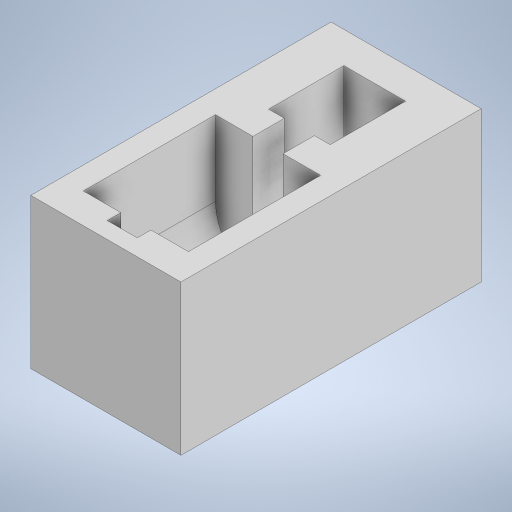
# Autodesk Inventor part: dcmotor_housing
Saved by Autodesk Inventor 2023 (Build 270158000, 158)
## iProperties
Created: 2023-03-20
Part Number: dcmotor_housing
Material: Generic
Document SubType Name: Modeling
Designer: caleb
Density: 1 g/cm^3
Appearance: Default
Author: caleb
Autodesk Inventor part; units mm, degrees
sketch "Sketch1" plane through (0, 0, 0) normal (0, 1, 0) x (-1, 0, 0)
  line L0 (0, 0) -> (50, 0)
  line L1 (50, 0) -> (50, -100)
  line L2 (50, -100) -> (0, -100)
  line L3 (0, -100) -> (0, 0)
  line L4 (25, 0) -> (25, -100)
  line L5 (7.5, -54) -> (7.5, -10)
  line L6 (7.5, -10) -> (42.5, -10)
  line L7 (42.5, -10) -> (42.5, -54)
  line L8 (42.5, -54) -> (7.5, -54)
  line L9 (7.5, -54) -> (42.5, -10) construction
  line L10 (7.5, -10) -> (42.5, -54) construction
  line L11 (7.5, -54) -> (51.5, -54) construction
  line L12 (14.75, -64.45) -> (14.75, -89.55)
  line L13 (14.75, -89.55) -> (35.25, -89.55)
  line L14 (35.25, -89.55) -> (35.25, -64.45)
  line L15 (35.25, -64.45) -> (14.75, -64.45)
  line L16 (14.75, -64.45) -> (35.25, -89.55) construction
  line L17 (14.75, -89.55) -> (35.25, -64.45) construction
  line L18 (14.75, -64.45) -> (39.85, -64.45) construction
  line L19 (25, -10) -> (25, -15)
  line L20 (25, -10) -> (30, -10) construction
  line L21 (20, -20) -> (30, -20)
  line L22 (30, -20) -> (30, -10)
  line L23 (30, -10) -> (20, -10)
  line L24 (20, -10) -> (20, -20)
  line L25 (20, -20) -> (30, -10) construction
  line L26 (30, -20) -> (20, -10) construction
  line L27 (20, -20) -> (30, -20) construction
  line L28 (30, -15) -> (20, -15)
  point P0 (25, -32)
  point P1 (25, -77)
  point P2 (25, -54)
  point P3 (25, -77)
  dimension "d0" = 50
  dimension "d1" = 100
  dimension "d4" = 44
  dimension "d5" = 90
  dimension "d6" = 35
  dimension "d7" = 10
  dimension "d8" = 25.1
  dimension "d9" = 90
  dimension "d10" = 20.5
  dimension "d35" = 5
  dimension "d36" = 90
  dimension "d37" = 0
  constraints: 58 end point, 11 midpoint, 9 parallel, 5 horizontal, 4 equal length, 4 perpendicular, 3 point on line, 1 coincident, 1 collinear, 1 vertical
  measures "d0" distance of L1.end L2.end
  measures "d1" distance of L0.end L1.end
  measures "d4" distance of L5.start L5.end
  measures "d5" angle of L11 L5
  measures "d6" distance of L5.end L6.end
  measures "d7" distance between parallel lines of L6 L0
  measures "d8" distance of L12.start L12.end
  measures "d9" angle of L12 L18
  measures "d10" distance of L13.end L12.end
  measures "d35" distance of L19.start L19.end
  measures "d36" angle of L19 L20
  measures "d37" distance between parallel lines of L21 L27
extrude "Extrusion1" add sketch "Sketch1" against normal blind 50
ref_plane "Work Plane3" through (-14.75, 0, -89.55) normal (0, 0, -1) x (-1, 0, 0)
ref_plane "Work Plane4" through (-7.5, 0, -54) normal (0, 0, -1) x (-1, 0, 0)
sketch "Sketch3" plane through (-14.75, 0, -89.55) normal (0, 0, -1) x (-1, 0, 0)
  line L0 (35.25, 0) -> (-14.75, 0) projected
  line L1 (35.25, 0) -> (35.25, -50) projected
  line L2 (-14.75, -50) -> (35.25, -50) projected
  line L3 (-14.75, 0) -> (-14.75, -50) projected
  circle A0 centre (10.25, -25) radius 10.1
  line L4 (20.35, -35.1) -> (20.35, -14.9)
  line L5 (20.35, -14.9) -> (0.15, -14.9)
  line L6 (0.15, -14.9) -> (0.15, -35.1)
  line L7 (0.15, -35.1) -> (20.35, -35.1)
  line L8 (20.35, -35.1) -> (0.15, -14.9) construction
  line L9 (20.35, -14.9) -> (0.15, -35.1) construction
  line L10 (20.35, -35.1) -> (40.55, -35.1) construction
  point P0 (10.25, -35.1)
  point P1 (0.15, -25)
  point P2 (20.35, -25)
  dimension "d18" = 20.2
  dimension "d21" = 90
  constraints: 14 end point, 2 midpoint, 2 parallel, 2 perpendicular, 1 centre point, 1 coincident, 1 horizontal
  measures "d18" diameter of A0
  measures "d21" angle of L10 L4
ref_plane "Work Plane5" through (-14.75, 0, -64.45) normal (0, 0, -1) x (-1, 0, 0)
ref_plane "Work Plane6" through (-7.5, 0, -10) normal (0, 0, -1) x (-1, 0, 0)
ref_plane "Work Plane7" through (-35.1, -35.1, -89.55) normal (0, 1, 0) x (1, 0, 0)
extrude "Extrusion5" cut sketch "Sketch1" against normal up to surface (35.1 mm away) contours L13 L12 L15 L4 | L4 L15 L14 L13
extrude "Extrusion6" add sketch "Sketch3" against normal up to surface (25.1 mm away) contours L4 L7 A0 | L7 L6 A0
sketch "Sketch4" plane through (-7.5, 0, -54) normal (0, 0, -1) x (-1, 0, 0)
  line L0 (42.5, 0) -> (-7.5, 0) projected
  line L1 (42.5, 0) -> (42.5, -50) projected
  line L2 (-7.5, -50) -> (42.5, -50) projected
  line L3 (-7.5, 0) -> (-7.5, -50) projected
  circle A0 centre (17.5, -25) radius 17.5
  line L4 (0, -42.5) -> (0, -7.5)
  line L5 (0, -7.5) -> (35, -7.5)
  line L6 (35, -7.5) -> (35, -42.5)
  line L7 (35, -42.5) -> (0, -42.5)
  line L8 (0, -42.5) -> (35, -7.5) construction
  line L9 (0, -7.5) -> (35, -42.5) construction
  line L10 (0, -42.5) -> (35, -42.5) construction
  point P0 (17.5, -42.5)
  point P1 (35, -25)
  point P2 (0, -25)
  dimension "d26" = 35
  dimension "d27" = 90
  constraints: 14 end point, 2 midpoint, 2 parallel, 2 perpendicular, 1 centre point, 1 coincident, 1 horizontal
  measures "d26" diameter of A0
  measures "d27" angle of L10 L4
ref_plane "Work Plane8" through (-7.5, -42.5, -54) normal (0, 1, 0) x (1, 0, 0)
extrude "Extrusion7" cut sketch "Sketch1" against normal up to surface (42.5 mm away) contours L6 L22 L28 L4 | L4 L28 L24 L6 | L28 L22 L21 L4 | L4 L21 L24 L28 | L24 L21 L4 L8 L5 L6 | L6 L7 L8 L4 L21 L22
extrude "Extrusion8" add sketch "Sketch4" against normal up to surface (44 mm away) contours L6 L7 A0 | L7 L4 A0
sketch "Sketch5" plane through (-14.75, 0, -64.45) normal (0, 0, -1) x (-1, 0, 0)
  line L0 (35.25, 0) -> (-14.75, 0) projected
  line L1 (35.25, 0) -> (35.25, -50) projected
  line L2 (-14.75, -50) -> (35.25, -50) projected
  line L3 (-14.75, 0) -> (-14.75, -50) projected
  circle A0 centre (10.25, -25) radius 5
  dimension "d32" = 10
  constraints: 1 centre point, 1 coincident
  measures "d32" diameter of A0
extrude "Extrusion9" cut sketch "Sketch5" against normal blind 59 contours A0
extrude "Extrusion10" cut sketch "Sketch1" against normal through all contours L6 L22 L28 L4 | L4 L28 L24 L6
ref_plane "Work Plane9" through (-25, -25, -64.45) normal (0, 1, 0) x (1, 0, 0)
sketch "Sketch6" plane through (-25, -25, -64.45) normal (0, 1, 0) x (1, 0, 0)
  line L0 (-5, 0) -> (-5, -10.45) projected
  line L1 (-5, 0) -> (5, 0) projected
  line L2 (5, -10.45) -> (-5, -10.45) projected
  line L3 (5, -10.45) -> (-5, -10.45) projected
  line L4 (-5, -10.45) -> (5, -10.45)
  line L5 (5, -10.45) -> (5, 0)
  line L6 (5, 0) -> (-5, 0)
  line L7 (-5, 0) -> (-5, -10.45)
  line L8 (-5, -59) -> (5, -59) projected
  line L9 (-5, -54.45) -> (-5, -59) projected
  line L10 (5, -54.45) -> (5, -59) projected
  line L11 (-5, -54.45) -> (5, -54.45) projected
  line L12 (5, -54.45) -> (-5, -54.45)
  line L13 (-5, -54.45) -> (-5, -59)
  line L14 (-5, -59) -> (5, -59)
  line L15 (5, -59) -> (5, -54.45)
  point P0 (25, -64.45)
  constraints: 16 end point, 4 parallel, 2 horizontal, 2 perpendicular
extrude "Extrusion11" cut sketch "Sketch6" along normal through all
sketch "Sketch7" plane through (0, -50, 0) normal (0, -1, 0) x (1, 0, 0)
  line L0 (-50, -100) -> (0, -100) projected
  line L1 (-25, -100) -> (-25, -80)
  line L2 (-25, -80) -> (-35, -80)
  line L3 (-35, -80) -> (-35, -85)
  line L4 (-35, -85) -> (-25, -85)
  line L5 (-25, -85) -> (-25, -80)
  line L6 (-35, -85) -> (-15, -85)
  line L7 (-15, -85) -> (-15, -80)
  line L8 (-15, -80) -> (-35, -80)
  line L9 (-35, -80) -> (-35, -85)
  point P0 (0, 0)
  dimension "d42" = 20
  dimension "d43" = 10
  dimension "d44" = 5
  dimension "d45" = 20
  constraints: 18 end point, 4 parallel, 2 horizontal, 2 perpendicular, 1 midpoint, 1 point on line, 1 vertical
  measures "d42" distance of L1.start L1.end
  measures "d43" distance of L4.end L3.end
  measures "d44" distance of L3.end L2.end
  measures "d45" distance of L8.end L7.end
extrude "Extrusion12" add sketch "Sketch7" along normal blind 10
body "Solid1"
